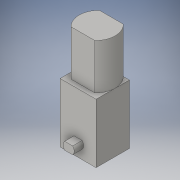
# Autodesk Inventor part: Motor
Saved by Autodesk Inventor 2016 (Build 200138000, 138)
## iProperties
Created: 2017-09-11
Part Number: Motor
Material: Generic
Document SubType Name: Modeling
Designer: student
Density: 1 g/cm^3
Appearance: Default
Author: student
Autodesk Inventor part; units mm, degrees
ref_plane "YZ Plane" through (0, 0, 0) normal (1, 0, 0) x (0, 1, 0)
ref_plane "XZ Plane" through (0, 0, 0) normal (0, 1, 0) x (-1, 0, 0)
ref_plane "XY Plane" through (0, 0, 0) normal (0, 0, 1) x (1, 0, 0)
sketch "Sketch1" plane through (0, 0, 0) normal (0, 0, 1) x (1, 0, 0)
  line L0 (0, 0) -> (22.5044, 0)
  line L1 (22.5044, 0) -> (22.5044, 37.084)
  line L2 (22.5044, 37.084) -> (0, 37.084)
  line L3 (0, 37.084) -> (0, 0)
  dimension "d0" = 22.5044
  dimension "d1" = 37.084
  constraints: 8 end point, 2 parallel, 1 horizontal, 1 perpendicular
  measures "d0" distance of L2.end L1.end
  measures "d1" distance of L0.end L1.end
extrude "Extrusion1" add sketch "Sketch1" along normal blind 20.828
sketch "Sketch2" plane through (0, 37.084, 0) normal (0, 1, 0) x (1, 0, 0)
  line L0 (0, 0) -> (22.5044, 0) projected
  line L1 (11.2522, 0) -> (11.2522, -8.89)
  line L2 (11.2522, -8.89) -> (11.2522, -17.78)
  line L3 (11.2522, -17.78) -> (3.8354, -17.78)
  line L4 (11.2522, -17.78) -> (18.669, -17.78)
  arc A0 (3.8354, 0) -> (3.8354, -17.78) centre (12.2207, -8.89) ccw
  line L5 (0, 0) -> (0, -20.828) projected
  arc A1 (18.669, -17.78) -> (18.669, 0) centre (10.2837, -8.89) ccw
  line L6 (22.5044, 0) -> (22.5044, -20.828) projected
  line L7 (3.8354, 0) -> (18.669, 0)
  dimension "d4" = 8.89
  dimension "d5" = 8.89
  dimension "d6" = 7.4168
  dimension "d7" = 7.4168
  constraints: 10 end point, 4 point on circle, 2 centre point, 2 horizontal, 2 point on line, 2 tangent, 2 vertical, 1 collinear, 1 midpoint
  measures "d4" distance of L1.start L1.end
  measures "d5" distance of L1.end L2.end
  measures "d6" distance of L2.end L3.end
  measures "d7" distance of L2.end L4.end
extrude "Extrusion2" add sketch "Sketch2" along normal blind 28.3718 contours L0 L1 L2 L3 A0 | L0 A1 L4 L2 L1
sketch "Sketch3" plane through (0, 0, 20.828) normal (0, 0, 1) x (1, 0, 0)
  line L0 (22.5044, 0) -> (22.5044, 37.084) projected
  line L1 (0, 0) -> (22.5044, 0) projected
  line L2 (13.7541, 10.3759) -> (8.7503, 10.3759)
  line L3 (8.7503, 5.5753) -> (13.7541, 5.5753)
  line L4 (13.7541, 10.3759) -> (8.7503, 5.5753) construction
  line L5 (8.7503, 10.3759) -> (13.7541, 5.5753) construction
  line L6 (0, 37.084) -> (0, 0) projected
  arc A0 (13.7541, 5.5753) -> (13.7541, 10.3759) centre (11.2521, 7.9756) ccw
  arc A1 (8.7503, 10.3759) -> (8.7503, 5.5753) centre (11.2517, 7.9756) ccw
  point P0 (11.2522, 7.9756)
  dimension "d21" = 5.0038
  dimension "d22" = 4.8006
  constraints: 8 end point, 4 point on circle, 2 centre point, 1 horizontal, 1 parallel
  measures "d21" distance of L3.end L3.start
  measures "d22" distance of L3.start L2.end
extrude "Extrusion3" add sketch "Sketch3" along normal blind 5.8928
sketch "Sketch4" plane through (0, 0, 0) normal (0, 0, -1) x (-1, 0, 0)
  circle A0 centre (-11.2521, 18.9738) radius 3.4672
  point P0 (0, 0)
  constraints: 1 centre point
body "Solid1"
